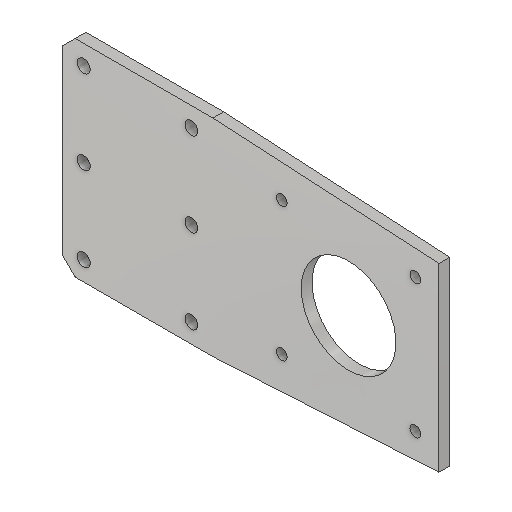
# Autodesk Inventor part: LC_ALU_3mm_X_axis_stepper_mount_plate
Saved by Autodesk Inventor 2025 (Build 290162010, 162A)
## iProperties
Created: 2018-07-10
Part Number: LC_ALU_3mm_X_axis_stepper_mount_plate
Material: Aluminum 6061-AHC
Document SubType Name: Modeling
Designer: Andrzej
Density: 2.7 g/cm^3
Appearance: Aluminum - Polished
Author: Andrzej
Autodesk Inventor part; units mm, degrees
ref_plane "YZ Plane" through (0, 0, 0) normal (1, 0, 0) x (0, 1, 0)
ref_plane "XZ Plane" through (0, 0, 0) normal (0, 1, 0) x (-1, 0, 0)
ref_plane "XY Plane" through (0, 0, 0) normal (0, 0, 1) x (1, 0, 0)
sketch "Sketch1" plane through (0, 0, 0) normal (0, 0, 1) x (1, 0, 0)
  line L0 (-21.273, 9.4908) -> (-21.273, -38.5092)
  line L1 (-21.273, -38.5092) -> (13.727, -38.5092)
  line L2 (66.227, -35.5092) -> (66.227, 6.4908)
  line L3 (-21.273, 9.4908) -> (13.727, 9.4908)
  line L4 (13.727, 9.4908) -> (13.727, 6.4908)
  line L5 (13.727, 6.4908) -> (66.227, 6.4908)
  line L6 (13.727, 6.4908) -> (13.727, -38.5092)
  line L7 (66.227, -35.5092) -> (13.727, -35.5092)
  line L8 (13.727, -38.5092) -> (66.227, -35.5092)
  line L9 (66.227, 6.4908) -> (13.727, 9.4908)
  point P0 (0, 0)
  point P1 (-16.273, 4.9908)
  point P2 (-16.273, -14.5092)
  point P3 (-16.273, -34.0092)
  point P4 (8.727, 4.9908)
  point P5 (8.727, -14.5092)
  point P6 (8.727, -34.0092)
  point P7 (29.727, 0.9908)
  point P8 (29.727, -30.0092)
  point P9 (60.727, -30.0092)
  point P10 (60.727, 0.9908)
  point P11 (45.227, -14.5092)
  dimension "d0" = 48
  dimension "d2" = 42
  dimension "d3" = 35
  dimension "d4" = 5
  dimension "d5" = 5
  dimension "d6" = 4.5
  dimension "d7" = 4.5
  dimension "d8" = 24
  dimension "d9" = 31
  dimension "d10" = 31
  dimension "d13" = 15.5
  dimension "d14" = 15.5
  dimension "d44" = 5.5
  dimension "d45" = 87.5
  dimension "d46" = 5.5
  dimension "d47" = 3
  dimension "d52" = 52.5
  constraints: 20 end point, 6 vertical alignment, 5 horizontal alignment, 5 perpendicular, 2 vertical, 1 horizontal, 1 point on line
  measures "d0" distance of L0.start L0.end
  measures "d2" distance of L2.start L2.end
  measures "d3" distance of L0.start L3.end
  measures "d4" distance from line of L0 point (-16.273, 4.991)
  measures "d5" distance from line of L4 point (8.727, 4.991)
  measures "d6" distance from line of L3 point (-16.273, 4.991)
  measures "d7" distance from line of L1 point (-16.273, -34.009)
  measures "d8" distance from line of L3 point (-16.273, -14.509)
  measures "d9" distance of point (29.727, -30.009) point (29.727, 0.991)
  measures "d10" distance of point (29.727, 0.991) point (60.727, 0.991)
  measures "d13" horizontal distance of point (29.727, 0.991) point (45.227, -14.509)
  measures "d14" horizontal distance of point (29.727, -30.009) point (45.227, -14.509)
  measures "d44" distance from line of L2 point (60.727, -30.009)
  measures "d45" distance between parallel lines of L0 L2
  measures "d46" distance from line of L7 point (60.727, -30.009)
  measures "d47" distance between parallel lines of L1 L7
  measures "d52" distance between parallel lines of L2 L6
extrude "Extrusion1" add sketch "Sketch1" along normal blind 2.5
hole "Hole1" at (-16.273, 4.9908, 0) at (-16.273, -14.5092, 0) at (-16.273, -34.0092, 0) at (8.727, 4.9908, 0) at (8.727, -14.5092, 0) at (8.727, -34.0092, 0) direction (0, 0, 1) diameter 3 end through all
hole "Hole2" at (29.727, 0.9908, 0) at (29.727, -30.0092, 0) at (60.727, -30.0092, 0) at (60.727, 0.9908, 0) direction (0, 0, 1) diameter 2.5 end through all
hole "Hole3" at (45.227, -14.5092, 0) direction (0, 0, 1) diameter 22 end through all
chamfer "Chamfer3" distance 3 angle 45 2 edges at (-21.273, -38.5092, 1.25) (-21.273, 9.4908, 1.25)
equation "\"d5\" = d4"
equation "\"d10\" = d9"
equation "\"d13\" = 0.5 * d9"
equation "\"d14\" = d13"
equation "\"d46\" = d44"
equation "\"d47\" = -0.5 * d2 + 0.5 * d0"
body "Solid1"
